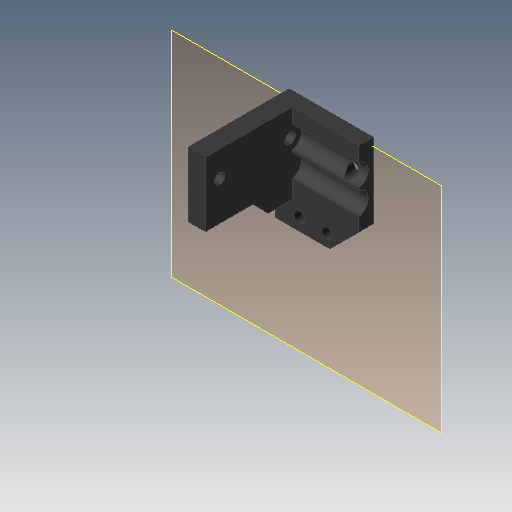
# Autodesk Inventor part: cellSTORM_alviumadapter
Saved by Autodesk Inventor 2019.4 (Build 234330000, 330)
## iProperties
Created: 2020-06-15
Part Number: cellSTORM_alviumadapter
Material: Generic
Document SubType Name: Modeling
Designer: diederichbenedict
Density: 1 g/cm^3
Appearance: Default
Author: diederichbenedict
Autodesk Inventor part; units mm, degrees
ref_plane "YZ Plane" through (0, 0, 0) normal (1, 0, 0) x (0, 1, 0)
ref_plane "XZ Plane" through (0, 0, 0) normal (0, 1, 0) x (-1, 0, 0)
ref_plane "Work Plane1" through (0, 0, 0) normal (0, 0, 1) x (1, 0, 0)
sketch "Sketch1" plane through (0, 0, 0) normal (0, 0, 1) x (1, 0, 0)
  circle A0 centre (2.6061, 6.2821) radius 1.5 construction
  circle A1 centre (22.6061, 6.2821) radius 1.5 construction
  line L0 (-2.6427, 15.6321) -> (-2.6427, -2.7179) construction
  line L1 (-2.6427, -2.7179) -> (30.1061, -2.7179) construction
  line L2 (30.1061, -2.7179) -> (30.1061, -39.6443) construction
  line L3 (30.1061, -39.6443) -> (66.9651, 7.5331) construction
  line L4 (66.9651, 7.5331) -> (66.9651, 15.6321) construction
  line L5 (66.9651, 15.6321) -> (-2.6427, 15.6321) construction
  circle A2 centre (12.3511, 11.6321) radius 1.45 construction
  circle A3 centre (41.9344, -5.4679) radius 1.45 construction
  circle A4 centre (34.1061, -5.4679) radius 1.45 construction
  circle A5 centre (54.6178, 11.6321) radius 1.45 construction
  circle A6 centre (-0.6427, 11.6823) radius 1.45 construction
  circle A7 centre (29.5857, 11.6321) radius 1.45 construction
  circle A8 centre (51.7579, -5.4342) radius 1.45 construction
  circle A9 centre (34.1061, -24.4536) radius 1.45 construction
  circle A10 centre (47.169, 11.6321) radius 1.45 construction
  line L6 (-7.0605, -146.6377) -> (1.2368, -137.4227) construction
  line L7 (-28.8718, -126.9987) -> (-20.5745, -117.7837) construction
  line L8 (32.1612, -8.9378) -> (42.8353, -8.9378)
  line L9 (42.8353, -8.9378) -> (51.0915, -0.6816)
  line L10 (51.0915, -0.6816) -> (51.0915, 15.6321)
  line L11 (32.1612, -8.9378) -> (32.1612, 15.6321)
  line L12 (32.1612, 15.6321) -> (51.0915, 15.6321)
  circle A11 centre (34.1061, -5.4679) radius 1.55
  circle A12 centre (41.9344, -5.4679) radius 1.55
  circle A13 centre (47.169, 11.6321) radius 1.55
  line L13 (32.1612, 15.6321) -> (51.0915, 15.6321)
  line L14 (51.0915, 15.6321) -> (51.0915, 20.6321)
  line L15 (51.0915, 20.6321) -> (32.1612, 20.6321)
  line L16 (32.1612, 20.6321) -> (32.1612, 15.6321)
  point P0 (0, 0)
  dimension "d0" = 135
  dimension "d1" = 3.1
  dimension "d2" = 3.1
  dimension "d3" = 3.1
  dimension "d16" = 5
  constraints: 18 end point, 3 centre point, 3 coincident, 2 horizontal, 2 parallel, 2 perpendicular, 1 collinear, 1 midpoint, 1 point on line
  measures "d0" angle of L9 L8
  measures "d1" diameter of A11
  measures "d2" diameter of A12
  measures "d3" diameter of A13
  measures "d16" distance of L14.end L13.end
extrude "Extrusion1" add sketch "Sketch1" along normal blind 4
sketch "Sketch2" plane through (32.1612, -8.9378, 0) normal (-1, 0, 0) x (0, 0, 1)
  line L0 (0, 0) -> (0, 29.5699) projected
  line L1 (0, 0) -> (4, 0) projected
  line L2 (4, 29.5699) -> (4, 0) projected
  line L3 (10.8285, 6.8285) -> (15.2199, 11.2199)
  line L4 (15.2199, 11.2199) -> (28.65, 11.2199)
  line L5 (28.65, 11.2199) -> (28.65, 29.5699)
  line L6 (28.65, 29.5699) -> (0, 29.5699)
  line L7 (10.8285, 6.8285) -> (0, 6.8285)
  line L8 (0, 0) -> (0, 8.2562) projected
  line L9 (0, 29.5699) -> (4, 29.5699) projected
  ellipse E0 centre (24.65, -131.1602) end of major axis (23.05, -131.1602) minor radius 1.189 projected
  ellipse E1 centre (4.65, -131.1602) end of major axis (3.05, -131.1602) minor radius 1.189 projected
  point P0 (0, 8.9378)
  point P1 (0, 6.2199)
  dimension "d8" = 45
  constraints: 10 end point, 2 horizontal, 2 perpendicular, 1 point on line, 3 other
  measures "d8" angle of L2 L3
ref_plane "Work Plane2" through (27.2811, 2.682, 0.7251) normal (1, 0, 0) x (0, 1, 0)
extrude "Extrusion2" add sketch "Sketch2" along normal up to surface (4.8801 mm away) contours L0 L7 L2 L1 | L0 L6 L2 L7 | L2 L6 L5 L4 L3 L7
sketch "Sketch3" plane through (51.0915, -0.6816, 0) normal (1, 0, 0) x (0, 0, -1)
  circle A0 centre (-24.65, 13.9637) radius 1.5
  circle A1 centre (-4.65, 13.9637) radius 1.5
  ellipse E0 centre (-4.65, -139.4164) end of major axis (-3.05, -139.4164) minor radius 1.189 projected
  ellipse E1 centre (-24.65, -139.4164) end of major axis (-23.05, -139.4164) minor radius 1.189 projected
  point P0 (0, 0.6816)
  dimension "d17" = 3
  dimension "d18" = 3
  constraints: 2 centre point, 2 other
  measures "d17" diameter of A0
  measures "d18" diameter of A1
extrude "Extrusion3" cut sketch "Sketch3" against normal through all
sketch "Sketch4" plane through (51.0915, -0.6816, 0) normal (1, 0, 0) x (0, 0, -1)
  arc A0 (-4, 5.5016) -> (-4, 8.4257) centre (-4.65, 6.9637) ccw projected
  circle A1 centre (-4.65, 6.9637) radius 3.25
  arc A2 (-4, 12.6118) -> (-4, 15.3155) centre (-4.65, 13.9637) ccw projected
  circle A3 centre (-4.65, 13.9637) radius 3.2592
  point P0 (0, 0.6816)
  dimension "d13" = 6.5
  constraints: 2 centre point, 2 coincident
  measures "d13" diameter of A1
extrude "Extrusion4" cut sketch "Sketch4" against normal up to surface (18.9303 mm away)
body "Solid1"
